Autodesk Fusion 360 part; units mm, degrees
(part 2 of 2)
fillet "Fillet2'''" radius 16 2 edges at (10, -27.5, 30) (10, -27.5, -30) on bodies 15 in component "SideBracket_Light_DropIn"
fillet "Fillet2'''" radius 4 7 edges at (2.5, -10, -24) (2.5, -16, -30) (2.5, -10, 24) (2.5, -16, 30) (10, -15, 12.1) (10, -15, -12.1) (37.1463, -27.5, 17) on bodies 15 in component "SideBracket_Light_DropIn"
move_body "Move1''''''''" bodies 15 to x (1, 0, 0) y (0, 1, 0) z (0, 0, 1) at (0, -120, 0) in component "SideBracket_Light_DropIn"
chamfer "Chamfer5'''" distance 1 angle 45 10 edges at (24.8021, -150, 22.9115) (9.9098, -150, 29.6027) (3.1832, -150, 30) (51.9306, -150, -7.5147) (54.1, -150, 7.875) (53.7339, -150, 16.6339) (45.4523, -150, 17) (3.1832, -150, -30) (9.9098, -150, -29.6027) (29.6836, -150, -20.5738) on bodies 15 in component "SideBracket_Light_DropIn"
component "SideBracket_Heavy_" placed x (1, 0, 0) y (0, 1, 0) z (0, 0, 1) at (0, 0, 0)
component "Hanger_25ID_65W_" placed x (1, 0, 0) y (0, 1, 0) z (0, 0, 1) at (0, 0, 0)
component "SupportBracket_" placed x (1, 0, 0) y (0, 1, 0) z (0, 0, 1) at (0, -90, 0)
component "SideBracket_Light_" placed x (1, 0, 0) y (0, 1, 0) z (0, 0, 1) at (0, 0, 0)
component "Hanger_25ID_35W_" placed x (1, 0, 0) y (0, 1, 0) z (0, 0, 1) at (0, 0, 0)
component "Hanger_25ID_30W_" placed x (1, 0, 0) y (0, 1, 0) z (0, 0, 1) at (0, 0, 0)
component "Hanger_25ID_25W_" placed x (1, 0, 0) y (0, 1, 0) z (0, 0, 1) at (0, 0, 0)
component "Hanger_25ID_20W_" placed x (1, 0, 0) y (0, 1, 0) z (0, 0, 1) at (0, 0, 0)
component "HangerLabel_" placed x (1, 0, 0) y (0, 1, 0) z (0, 0, 1) at (0, 0, 0)
component "Hanger_Hook_20Spacer" placed x (1, 0, 0) y (0, 1, 0) z (0, 0, 1) at (0, 0, 0)
component "Hanger_Hook_Thin" placed x (1, 0, 0) y (0, 1, 0) z (0, 0, 1) at (0, 0, 0)
component "RingSpacer" placed x (1, 0, 0) y (0, 1, 0) z (0, 0, 1) at (0, 0, 0)
component "SideBracket_Heavy_ DropIn" placed x (1, 0, 0) y (0, 1, 0) z (0, 0, 1) at (0, 0, 80)
component "SupportBracket_ DropIn" placed x (1, 0, 0) y (0, 1, 0) z (0, 0, 1) at (0, -90, 80)
component "SideBracket_Light_DropIn" placed x (1, 0, 0) y (0, 1, 0) z (0, 0, 1) at (0, 0, 80)
equation "XY_Tolerance = 0.2 mm"
equation "Z_Tolerance = 0.2 mm"
equation "Wall_Thickness = 0.4 mm"
equation "Layer_Height = 0.2 mm"
equation "M3Hole_wClearance = 3.2 mm"
equation "M3Hole_wSelfTapping = 2.8 mm"
equation "d28 = M3Hole_wClearance"
equation "M3Hole_CounterSink = 1.8 mm"
equation "d60 = HangDepth"
equation "d93 = XY_Tolerance"
equation "d97 = SupportRodDia"
equation "d136 = WallOffset"
equation "d137 = SupportRodDia + XY_Tolerance"
equation "SupportRodDia = 20 mm"
equation "WallOffset = 40 mm"
equation "d169 = M3Hole_CounterSink"
equation "d169_1 = M3Hole_CounterSink"
equation "d169_1_1 = M3Hole_CounterSink"
equation "HangDepth = 50 mm" comment "50 & 30 are the standard sizes i used"
equation "d215 = XY_Tolerance"
equation "d216 = XY_Tolerance"
equation "d218 = XY_Tolerance"
equation "d219 = XY_Tolerance"
equation "d220 = LabelWidth"
equation "d229 = 1 mm + ( XY_Tolerance / 2 )"
equation "LabelWidth = 30 mm"
equation "d169_2 = M3Hole_CounterSink"
equation "d169_1_2 = M3Hole_CounterSink"
equation "d169_1_1_1 = M3Hole_CounterSink"
